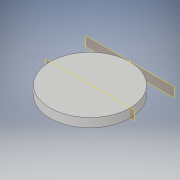
# Autodesk Inventor part: Lid
Saved by Autodesk Inventor 2017.2 (Build 212233000, 233)
## iProperties
Created: 2017-04-02
Part Number: Lid
Material: Generic
Document SubType Name: Modeling
Designer: steele
Density: 1 g/cm^3
Appearance: Default
Author: steele
Autodesk Inventor part; units mm, degrees
ref_plane "YZ Plane" through (0, 0, 0) normal (1, 0, 0) x (0, 1, 0)
ref_plane "XZ Plane" through (0, 0, 0) normal (0, 1, 0) x (-1, 0, 0)
sketch "Sketch1" plane through (0, 0, 0) normal (0, 1, 0) x (-1, 0, 0)
  circle A0 centre (0, 0) radius 57.15
  dimension "d0" = 114.3
  constraints: 1 centre point, 1 coincident
  measures "d0" diameter of A0
extrude "Extrusion1" add sketch "Sketch1" against normal blind 12.7
sketch "Sketch2" plane through (0, -12.7, 0) normal (0, -1, 0) x (1, 0, 0)
  circle A0 centre (0, 0) radius 53.975
  dimension "d3" = 107.95
  constraints: 1 centre point, 1 coincident
  measures "d3" diameter of A0
extrude "Extrusion2" cut sketch "Sketch2" against normal blind 9.525
ref_plane "Work Plane1" through (0, 0, -57.15) normal (0, 0, 1) x (1, 0, 0)
sketch "Sketch3" plane through (0, 0, -57.15) normal (0, 0, 1) x (1, 0, 0)
  point P0 (0, 0)
equation "\"d0\" = OutsideDiam"
equation "\"d1\" = Height"
equation "\"d3\" = InsideDiam"
equation "\"d4\" = Height - TopThickness"
equation "\"OutsideDiam\" = 114.3"
equation "\"InsideDiam\" = 107.95"
equation "\"Height\" = 12.7"
equation "\"TopThickness\" = 3.175"
body "Solid1"
